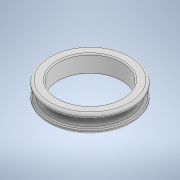
# Autodesk Inventor part: Poly belt pulley for 1 inchj sched 40 pvc
Saved by Autodesk Inventor 2020 (Build 240168000, 168)
## iProperties
Created: 2020-01-21
Part Number: Poly belt pulley for 1 inchj sched 40 pvc
Material: Generic
Document SubType Name: Modeling
Designer: JimAndVal
Density: 1 g/cm^3
Appearance: Default
Author: JimAndVal
## iProperties of the stored document _3DPrint.ipt
Created: 2020-01-22
Part Number: _3DPrint
Material: Generic
Document SubType Name: Modeling
Designer: JimAndVal
Density: 1 g/cm^3
Appearance: Default
Author: JimAndVal
Autodesk Inventor part; units mm, degrees
ref_plane "YZ Plane" through (0, 0, 0) normal (1, 0, 0) x (0, 1, 0)
ref_plane "XZ Plane" through (0, 0, 0) normal (0, 1, 0) x (-1, 0, 0)
ref_plane "XY Plane" through (0, 0, 0) normal (0, 0, 1) x (1, 0, 0)
sketch "Sketch1" plane through (0, 0, 0) normal (0, 0, 1) x (1, 0, 0)
  line L0 (0, 0) -> (0, 9.525)
  line L1 (0, 9.525) -> (20.955, 9.525)
  line L2 (20.955, 0) -> (0, 0)
  line L3 (22.225, 4.7625) -> (20.2311, 4.7625) construction
  arc A0 (20.2311, 7.239) -> (20.2311, 2.286) centre (20.2311, 4.7625) ccw
  line L4 (20.2311, 7.239) -> (21.717, 7.239)
  line L5 (20.2311, 2.286) -> (21.717, 2.286)
  arc A1 (22.225, 8.255) -> (20.955, 9.525) centre (20.955, 8.255) ccw
  arc A2 (20.955, 0) -> (22.225, 1.27) centre (20.955, 1.27) ccw
  line L6 (22.225, 8.255) -> (22.225, 7.747)
  line L7 (22.225, 1.778) -> (22.225, 1.27)
  arc A3 (21.717, 7.239) -> (22.225, 7.747) centre (21.717, 7.747) ccw
  arc A4 (22.225, 1.778) -> (21.717, 2.286) centre (21.717, 1.778) ccw
  point P0 (22.225, 9.525)
  dimension "d0" = 9.525
  dimension "d1" = 22.225
  dimension "d2" = 1.9939
  dimension "d3" = 1.27
  dimension "d4" = 0.508
  dimension "d12" = 2.286
  dimension "d13" = 2.286
  constraints: 16 end point, 11 tangent, 10 point on circle, 8 perpendicular, 5 centre point, 2 equal radius, 1 coincident, 1 horizontal, 1 point on line, 1 vertical
  measures "d0" distance of L0.start L0.end
  measures "d1" distance of L0.end point (22.225, 9.525)
  measures "d2" distance of L3.start L3.end
  measures "d3" radius of A1
  measures "d4" radius of A3
  measures "d12" distance between parallel lines of L1 L4
  measures "d13" distance between parallel lines of L2 L5
revolve "Revolution1" add sketch "Sketch1" angle 360 about axis through (0, 0, 0) along (0, 1, 0)
sketch "Sketch2" plane through (0, 9.525, 0) normal (0, 1, 0) x (1, 0, 0)
  circle A0 centre (0, 0) radius 16.8275
  dimension "d6" = 33.655
  constraints: 1 centre point, 1 coincident
  measures "d6" diameter of A0
extrude "Extrusion1" cut sketch "Sketch2" against normal through all
fillet "Fillet1" radius 0.635 1 edges at (-16.8275, 9.525, 0)
fillet "Fillet2" radius 0.635 1 edges at (-16.8275, 0, 0)
body "Solid1"
